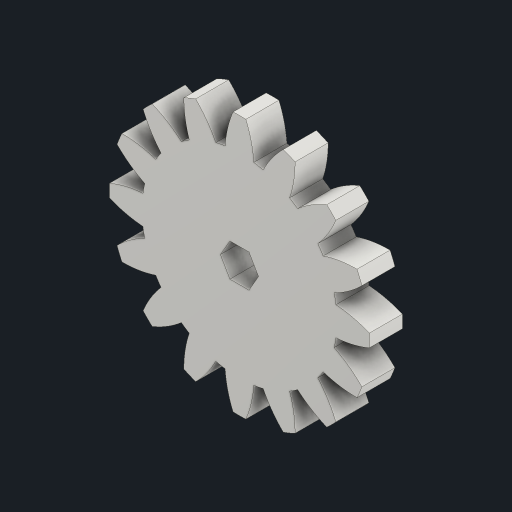
# Autodesk Inventor part: Spur Gear1
Saved by Autodesk Inventor 2024.3 (Build 283343000, 343)
## iProperties
CustomPartVersion: 1
Created: 2024-06-29
Part Number: Spur Gear1
Material: Steel
Document SubType Name: Modeling
Designer: Niler
Categories: <?xml version="1.0" encoding="UTF-16"?> <MemberInstance><Categories><FamilyTemplate><FamilyTemplateParameter ValueType="xs:double" Id="1" ObjectReferenceKey="da_z" ObjectType="kUserParameterObject"/><FamilyTemplateParameter ValueType="xs:double" Id="2" ObjectReferenceKey="da_b" ObjectType="kUserParameterObject"/><FamilyTemplateParameter ValueType="xs:double" Id="3" ObjectReferenceKey="da_beta" ObjectType="kUserParameterObject"/><FamilyTemplateParameter ValueType="xs:double" Id="4" ObjectReferenceKey="da_da" ObjectType="kUserParameterObject"/><FamilyTemplateParameter ValueType="xs:double" Id="5" ObjectReferenceKey="da_aw" ObjectType="kUserParameterObject"/><FamilyTemplateParameter ValueType="xs:string" Id="6" ObjectReferenceKey="EAIAABAAAACIAQAAAAAAAIAAAAAAAAAA" ObjectType="83910656" SubObjectId="SurfaceGeometry"/></FamilyTemplate><ParamToTemplateMap><ParamToTemplate CategoryParameter="//CategoryParameter[@InternalName='046C89C9-8512-4d59-83FE-43B91F4F132A']" TemplateParameter="1"/><ParamToTemplate CategoryParameter="//CategoryParameter[@InternalName='2552DF32-E462-4b46-AEBF-C6C7768E72AC']" TemplateParameter="2"/><ParamToTemplate CategoryParameter="//CategoryParameter[@InternalName='C9EE641D-15FC-4fae-A226-E94C4372FDD7']" TemplateParameter="3"/><ParamToTemplate><ParamToTemplate CategoryParameter="//CategoryParameter[@InternalName='00B6519A-459B-49c7-AD84-2E56D39A5744']" ConstantValue="0.000000"/></ParamToTemplate><ParamToTemplate><ParamToTemplate CategoryParameter="//CategoryParameter[@InternalName='04B31F0E-C7A6-4894-AA32-9629BEFACF47']" ConstantValue="1.000000"/></ParamToTemplate><ParamToTemplate><ParamToTemplate CategoryParameter="//CategoryParameter[@InternalName='43CBEC2E-7847-49e7-A936-2F7889FCB2D9']" ConstantValue="0.250000"/></ParamToTemplate><ParamToTemplate><ParamToTemplate CategoryParameter="//CategoryParameter[@InternalName='B1EFC894-105D-4ebd-86BF-FA20ED196853']" ConstantValue="0.350000"/></ParamToTemplate><ParamToTemplate><ParamToTemplate CategoryParameter="//CategoryParameter[@InternalName='51175063-3D10-4879-93E8-6246FE8B403D']" ConstantValue="2060000000.000000"/></ParamToTemplate><ParamToTemplate><ParamToTemplate CategoryParameter="//CategoryParameter[@InternalName='A3A52E27-4454-46a9-B0BD-C932399B70AF']" ConstantValue="0.300000"/></ParamToTemplate><ParamToTemplate><ParamToTemplate CategoryParameter="//CategoryParameter[@InternalName='91B76062-C214-41d9-B1B9-14D2AB99603D']" ConstantValue="0.350000"/></ParamToTemplate><ParamToTemplate><ParamToTemplate CategoryParameter="//CategoryParameter[@InternalName='374E806E-8B8A-4dda-A9AA-1039D6500AD2']" ConstantValue="2.857143"/></ParamToTemplate><ParamToTemplate><ParamToTemplate CategoryParameter="//CategoryParameter[@InternalName='2D373A89-B862-43d6-8D0B-0CBF12AB9F6C']" ConstantValue="0.349066"/></ParamToTemplate><ParamToTemplate CategoryParameter="//CategoryParameter[@InternalName='37777632-D6A2-4fac-9D53-DB8ACD95C989']" TemplateParameter="4"/><ParamToTemplate CategoryParameter="//CategoryParameter[@InternalName='FD1017F1-B727-4f7e-9707-0F86F1FF9423']" TemplateParameter="5"/><ParamToTemplate><ParamToTemplate CategoryParameter="//CategoryParameter[@InternalName='9E1B4470-B2D3-4ff1-B813-535BB4CDF51A']" ConstantValue="3520000.000000"/></ParamToTemplate><ParamToTemplate><ParamToTemplate CategoryParameter="//CategoryParameter[@InternalName='F8452263-BFF6-458c-9FB1-07C4B99E95CD']" ConstantValue="11400000.000000"/></ParamToTemplate><ParamToTemplate><ParamToTemplate CategoryParameter="//CategoryParameter[@InternalName='3E3BB259-FD49-497f-8171-6EBC954A3479']" ConstantValue="2.000000"/></ParamToTemplate><ParamToTemplate CategoryParameter="//CategoryParameter[@InternalName='27C3BAF2-7550-4e4b-AE2C-0DB134B7D9B7']" TemplateParameter="6"/></ParamToTemplateMap><Category DisplayName="Gear" InternalName="DC85795E-93AB-48d5-8EEE-5A27447B64BD" Mnemonic="Gear"><CategoryParameter DisplayName="z" InternalName="046C89C9-8512-4d59-83FE-43B91F4F132A" Mnemonic="z"/><CategoryParameter DisplayName="b" InternalName="2552DF32-E462-4b46-AEBF-C6C7768E72AC" Mnemonic="b"/><CategoryParameter DisplayName="||b|" InternalName="C9EE641D-15FC-4fae-A226-E94C4372FDD7" Mnemonic="beta"/><CategoryParameter DisplayName="x" InternalName="00B6519A-459B-49c7-AD84-2E56D39A5744" Mnemonic="x"/><CategoryParameter DisplayName="a*" InternalName="04B31F0E-C7A6-4894-AA32-9629BEFACF47" Mnemonic="a"/><CategoryParameter DisplayName="c*" InternalName="43CBEC2E-7847-49e7-A936-2F7889FCB2D9" Mnemonic="c"/><CategoryParameter DisplayName="r|.f|*" InternalName="B1EFC894-105D-4ebd-86BF-FA20ED196853" Mnemonic="rf"/><CategoryParameter DisplayName="E" InternalName="51175063-3D10-4879-93E8-6246FE8B403D" Mnemonic="E"/><CategoryParameter DisplayName="||m|" InternalName="A3A52E27-4454-46a9-B0BD-C932399B70AF" Mnemonic="mi"/><Category DisplayName="SpurGear" InternalName="26C5A22E-A91E-4dfd-A3B3-23CCAFAE1764" Mnemonic="SpurGear"><CategoryParameter DisplayName="m" InternalName="91B76062-C214-41d9-B1B9-14D2AB99603D" Mnemonic="m"/><CategoryParameter DisplayName="P" InternalName="374E806E-8B8A-4dda-A9AA-1039D6500AD2" Mnemonic="PP"/><CategoryParameter DisplayName="||a|" InternalName="2D373A89-B862-43d6-8D0B-0CBF12AB9F6C" Mnemonic="alpha"/><CategoryParameter DisplayName="d|.a|" InternalName="37777632-D6A2-4fac-9D53-DB8ACD95C989" Mnemonic="da"/><CategoryParameter DisplayName="a|.w|" InternalName="FD1017F1-B727-4f7e-9707-0F86F1FF9423" Mnemonic="aw"/><CategoryParameter DisplayName="||s||.Flim|" InternalName="9E1B4470-B2D3-4ff1-B813-535BB4CDF51A" Mnemonic="sFlim"/><CategoryParameter DisplayName="||s||.Hlim|" InternalName="F8452263-BFF6-458c-9FB1-07C4B99E95CD" Mnemonic="sHlim"/><CategoryParameter DisplayName="type" InternalName="3E3BB259-FD49-497f-8171-6EBC954A3479" Mnemonic="type"/><CategoryParameter DisplayName="PitchDiameter" InternalName="27C3BAF2-7550-4e4b-AE2C-0DB134B7D9B7" Mnemonic="IDS_PITCHDIAM"/></Category></Category></Categories></MemberInstance>
Density: 1 g/cm^3
Appearance: Steel
Author: Niler
Autodesk Inventor part; units mm, degrees
ref_plane "YZ Plane" through (0, 0, 0) normal (1, 0, 0) x (0, 1, 0)
ref_plane "XZ Plane" through (0, 0, 0) normal (0, 1, 0) x (-1, 0, 0)
ref_plane "XY Plane" through (0, 0, 0) normal (0, 0, 1) x (1, 0, 0)
sketch "Sketch1" plane through (0, 0, 0) normal (0, 0, 1) x (1, 0, 0)
  circle A0 centre (0, 0) radius 31.4721
  dimension "d0" = 62.9442
  constraints: 1 centre point
  measures "d0" diameter of A0
extrude "Extrusion1" add sketch "Sketch1" along normal blind 10
ref_plane "Work Plane2" through (0, 0, 5) normal (0, 0, 1) x (1, 0, 0)
sketch "Sketch2" plane through (0, 0, 0) normal (0, 0, -1) x (-1, 0, 0)
  circle A0 centre (0, 0) radius 31.4721 projected
  circle A1 centre (0, 0) radius 28
  dimension "d3" = 56
  constraints: 1 centre point, 1 coincident
  measures "d3" diameter of A1
surface extrude "Pitch Diameter" sketch "Sketch2" against normal through all shown no curves A1
ref_plane "Work Plane8" through (0, 0, 0) normal (0.9807853, 0.1950903, 0) x (0, 0, 1)
ref_plane "Work Plane9" through (0, 0, 0) normal (1, 0, 0) x (0, 1, 0)
spur gear teeth "Spur Gear" teeth 16 pitch diameter 56 tip diameter 62.9442 root diameter 47.25 face width 10 start plane through (0, 0, 0) normal (0, 0, -1) x (-1, 0, 0)
sketch "Sketch6" plane through (0, 0, 0) normal (0, 0, -1) x (-1, 0, 0)
  line L0 (4.6188, 0) -> (2.3094, -4)
  line L1 (2.3094, -4) -> (-2.3094, -4)
  line L2 (-2.3094, -4) -> (-4.6188, 0)
  line L3 (-4.6188, 0) -> (-2.3094, 4)
  line L4 (-2.3094, 4) -> (2.3094, 4)
  line L5 (2.3094, 4) -> (4.6188, 0)
  point P0 (0, 0)
  point P1 (0, 0)
  point P2 (0, -4)
  dimension "d62" = 8
  constraints: 12 end point, 1 coincident, 1 midpoint, 13 other
  measures "d62" distance from line of point (0, -4) L4
extrude "Extrusion4" cut sketch "Sketch6" against normal through all
sketch "Sketch7" plane through (0, 0, 10) normal (0, 0, 1) x (1, 0, 0)
  circle A0 centre (0, 0) radius 56.3298
  constraints: 1 centre point, 1 coincident
extrude "Extrusion5" cut sketch "Sketch7" against normal blind 2
sketch "Sketch3" plane through (0, 0, 10) normal (0, 0, 1) x (1, 0, 0)
  circle A0 centre (0, 0) radius 9
  circle A1 centre (0, 0) radius 5
  line L0 (-2, 0) -> (2, 0)
  line L1 (2, 0) -> (2, 6.5)
  line L2 (2, 6.5) -> (-2, 6.5)
  line L3 (-2, 6.5) -> (-2, 0)
  line L4 (2.15, 6.65) -> (2.15, -0.15)
  line L5 (2.15, -0.15) -> (-2.15, -0.15)
  line L6 (-2.15, -0.15) -> (-2.15, 6.65)
  line L7 (-2.15, 6.65) -> (2.15, 6.65)
  circle A2 centre (0, 0) radius 5.15
  point P0 (0, -5)
  point P1 (-2.15, 4.6797)
  point P2 (2.15, 4.6797)
  dimension "d50" = 10
  dimension "d49" = 18
  dimension "d52" = 11.5
  dimension "d53" = 4
  dimension "d54" = 0.15
  dimension "d55" = 0.15
  constraints: 16 end point, 4 parallel, 3 coincident, 2 centre point, 2 perpendicular, 2 vertical alignment, 1 horizontal, 1 midpoint, 5 other
  measures "d49" diameter of A0
  measures "d52" distance from line of point (0, -5) L2
  measures "d53" distance of L1.end L2.end
  measures "d54" distance between parallel lines of L1 L4
sketch "Sketch4" plane through (0, 0, 10) normal (0, 0, 1) x (1, 0, 0)
  line L0 (-2.15, 6.65) -> (2.15, 6.65) projected
  line L1 (2.15, 6.65) -> (2.15, 4.6797) projected
  arc A0 (-2.15, 4.6797) -> (2.15, 4.6797) centre (0, 0) ccw projected
  line L2 (-2.15, 4.6797) -> (-2.15, 6.65) projected
  arc A1 (-10.6026, -29.6324) -> (-5.7404, -22.917) centre (-28.6369, -11.4569) ccw projected
  arc A2 (-5.7404, -22.917) -> (-3.4665, -23.3693) centre (0, 0) ccw projected
  arc A3 (-3.4665, -23.3693) -> (-1.5443, -31.4342) centre (22.0727, -21.5436) ccw projected
  arc A4 (-1.5443, -31.4342) -> (1.5443, -31.4342) centre (0, 0) ccw projected
  arc A5 (1.5443, -31.4342) -> (3.4665, -23.3693) centre (-22.0727, -21.5436) ccw projected
  arc A6 (3.4665, -23.3693) -> (5.7404, -22.917) centre (0, 0) ccw projected
  arc A7 (5.7404, -22.917) -> (10.6026, -29.6324) centre (28.6369, -11.4569) ccw projected
  arc A8 (10.6026, -29.6324) -> (13.456, -28.4504) centre (0, 0) ccw projected
  arc A9 (13.456, -28.4504) -> (12.1457, -20.2638) centre (-12.1481, -28.3505) ccw projected
  arc A10 (12.1457, -20.2638) -> (14.0734, -18.9758) centre (0, 0) ccw projected
  arc A11 (14.0734, -18.9758) -> (21.1354, -23.3193) centre (30.8414, 0.3741) ccw projected
  arc A12 (21.1354, -23.3193) -> (23.3193, -21.1354) centre (0, 0) ccw projected
  arc A13 (23.3193, -21.1354) -> (18.9758, -14.0734) centre (-0.3741, -30.8414) ccw projected
  arc A14 (18.9758, -14.0734) -> (20.2638, -12.1457) centre (0, 0) ccw projected
  arc A15 (20.2638, -12.1457) -> (28.4504, -13.456) centre (28.3505, 12.1481) ccw projected
  arc A16 (28.4504, -13.456) -> (29.6324, -10.6026) centre (0, 0) ccw projected
  arc A17 (29.6324, -10.6026) -> (22.917, -5.7404) centre (11.4569, -28.6369) ccw projected
  arc A18 (22.917, -5.7404) -> (23.3693, -3.4665) centre (0, 0) ccw projected
  arc A19 (23.3693, -3.4665) -> (31.4342, -1.5443) centre (21.5436, 22.0727) ccw projected
  arc A20 (31.4342, -1.5443) -> (31.4342, 1.5443) centre (0, 0) ccw projected
  arc A21 (31.4342, 1.5443) -> (23.3693, 3.4665) centre (21.5436, -22.0727) ccw projected
  arc A22 (23.3693, 3.4665) -> (22.917, 5.7404) centre (0, 0) ccw projected
  arc A23 (22.917, 5.7404) -> (29.6324, 10.6026) centre (11.4569, 28.6369) ccw projected
  arc A24 (29.6324, 10.6026) -> (28.4504, 13.456) centre (0, 0) ccw projected
  arc A25 (28.4504, 13.456) -> (20.2638, 12.1457) centre (28.3505, -12.1481) ccw projected
  arc A26 (20.2638, 12.1457) -> (18.9758, 14.0734) centre (0, 0) ccw projected
  arc A27 (18.9758, 14.0734) -> (23.3193, 21.1354) centre (-0.3741, 30.8414) ccw projected
  arc A28 (23.3193, 21.1354) -> (21.1354, 23.3193) centre (0, 0) ccw projected
  arc A29 (21.1354, 23.3193) -> (14.0734, 18.9758) centre (30.8414, -0.3741) ccw projected
  arc A30 (14.0734, 18.9758) -> (12.1457, 20.2638) centre (0, 0) ccw projected
  arc A31 (12.1457, 20.2638) -> (13.456, 28.4504) centre (-12.1481, 28.3505) ccw projected
  arc A32 (13.456, 28.4504) -> (10.6026, 29.6324) centre (0, 0) ccw projected
  arc A33 (10.6026, 29.6324) -> (5.7404, 22.917) centre (28.6369, 11.4569) ccw projected
  arc A34 (5.7404, 22.917) -> (3.4665, 23.3693) centre (0, 0) ccw projected
  arc A35 (3.4665, 23.3693) -> (1.5443, 31.4342) centre (-22.0727, 21.5436) ccw projected
  arc A36 (1.5443, 31.4342) -> (-1.5443, 31.4342) centre (0, 0) ccw projected
  arc A37 (-1.5443, 31.4342) -> (-3.4665, 23.3693) centre (22.0727, 21.5436) ccw projected
  arc A38 (-3.4665, 23.3693) -> (-5.7404, 22.917) centre (0, 0) ccw projected
  arc A39 (-5.7404, 22.917) -> (-10.6026, 29.6324) centre (-28.6369, 11.4569) ccw projected
  arc A40 (-29.6324, -10.6026) -> (-28.4504, -13.456) centre (0, 0) ccw projected
  circle A41 centre (0, 0) radius 9.5
  arc A42 (-28.4504, -13.456) -> (-20.2638, -12.1457) centre (-28.3505, 12.1481) ccw projected
  arc A43 (-20.2638, -12.1457) -> (-18.9758, -14.0734) centre (0, 0) ccw projected
  arc A44 (-18.9758, -14.0734) -> (-23.3193, -21.1354) centre (0.3741, -30.8414) ccw projected
  arc A45 (-23.3193, -21.1354) -> (-21.1354, -23.3193) centre (0, 0) ccw projected
  arc A46 (-21.1354, -23.3193) -> (-14.0734, -18.9758) centre (-30.8414, 0.3741) ccw projected
  arc A47 (-14.0734, -18.9758) -> (-12.1457, -20.2638) centre (0, 0) ccw projected
  arc A48 (-12.1457, -20.2638) -> (-13.456, -28.4504) centre (12.1481, -28.3505) ccw projected
  arc A49 (-13.456, -28.4504) -> (-10.6026, -29.6324) centre (0, 0) ccw projected
  arc A50 (-13.456, 28.4504) -> (-12.1457, 20.2638) centre (12.1481, 28.3505) ccw projected
  arc A51 (-12.1457, 20.2638) -> (-14.0734, 18.9758) centre (0, 0) ccw projected
  arc A52 (-14.0734, 18.9758) -> (-21.1354, 23.3193) centre (-30.8414, -0.3741) ccw projected
  arc A53 (-21.1354, 23.3193) -> (-23.3193, 21.1354) centre (0, 0) ccw projected
  arc A54 (-23.3193, 21.1354) -> (-18.9758, 14.0734) centre (0.3741, 30.8414) ccw projected
  arc A55 (-18.9758, 14.0734) -> (-20.2638, 12.1457) centre (0, 0) ccw projected
  arc A56 (-20.2638, 12.1457) -> (-28.4504, 13.456) centre (-28.3505, -12.1481) ccw projected
  arc A57 (-28.4504, 13.456) -> (-29.6324, 10.6026) centre (0, 0) ccw projected
  arc A58 (-29.6324, 10.6026) -> (-22.917, 5.7404) centre (-11.4569, 28.6369) ccw projected
  arc A59 (-22.917, 5.7404) -> (-23.3693, 3.4665) centre (0, 0) ccw projected
  arc A60 (-23.3693, 3.4665) -> (-31.4342, 1.5443) centre (-21.5436, -22.0727) ccw projected
  arc A61 (-31.4342, 1.5443) -> (-31.4342, -1.5443) centre (0, 0) ccw projected
  arc A62 (-31.4342, -1.5443) -> (-23.3693, -3.4665) centre (-21.5436, 22.0727) ccw projected
  arc A63 (-23.3693, -3.4665) -> (-22.917, -5.7404) centre (0, 0) ccw projected
  arc A64 (-22.917, -5.7404) -> (-29.6324, -10.6026) centre (-11.4569, -28.6369) ccw projected
  arc A65 (-10.6026, 29.6324) -> (-13.456, 28.4504) centre (0, 0) ccw projected
  dimension "d58" = 19
  constraints: 1 centre point, 1 coincident
  measures "d58" diameter of A41
equation "\"d0\" = da_da"
equation "\"d1\" = da_b"
equation "\"d3\" = da_d"
equation "\"d16\" = da_aw"
equation "\"d43\" = da_aw"
equation "\"d46\" = da_aw"
equation "\"da_da\" = 62.944165"
equation "\"da_b\" = 10"
equation "\"da_d\" = 56"
equation "\"da_aw\" = 78"
body "Solid1"
body "Srf1"
